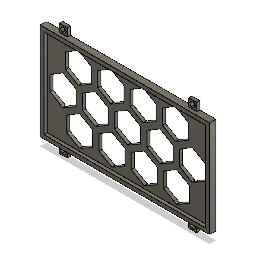
base (Autodesk Fusion 360 design; units mm, degrees)
Autodesk Fusion 360 part; units mm, degrees
sketch "Sketch1" plane through (0, 0, 0) normal (0, 0, 1) x (1, 0, 0)
  line L0 (0, 0) -> (0, 60)
  line L1 (0, 60) -> (10, 60)
  line L2 (10, 60) -> (10, 65)
  line L3 (10, 65) -> (15, 65)
  line L4 (15, 65) -> (15, 60)
  line L5 (15, 60) -> (90, 60)
  line L6 (90, 60) -> (90, 65)
  line L7 (90, 65) -> (95, 65)
  line L8 (95, 65) -> (95, 60)
  line L9 (95, 60) -> (105, 60)
  line L10 (105, 60) -> (105, 0)
  line L11 (105, 0) -> (95, 0)
  line L12 (95, 0) -> (95, -5)
  line L13 (95, -5) -> (90, -5)
  line L14 (90, -5) -> (90, 0)
  line L15 (90, 0) -> (15, 0)
  line L16 (15, 0) -> (15, -5)
  line L17 (15, -5) -> (10, -5)
  line L18 (10, -5) -> (10, 0)
  line L19 (10, 0) -> (0, 0)
  line L20 (10, 60) -> (15, 60) construction
  line L21 (12.5, 60) -> (12.5, 65) construction
  line L22 (90, 60) -> (95, 60) construction
  line L23 (92.5, 60) -> (92.5, 65) construction
  line L24 (90, 0) -> (95, 0) construction
  line L25 (92.5, 0) -> (92.5, -5) construction
  line L26 (10, 0) -> (15, 0) construction
  line L27 (12.5, 0) -> (12.5, -5) construction
  line L28 (13.366, 61) -> (14.2321, 62.5)
  line L29 (14.2321, 62.5) -> (13.366, 64)
  line L30 (13.366, 64) -> (11.634, 64)
  line L31 (11.634, 64) -> (10.7679, 62.5)
  line L32 (10.7679, 62.5) -> (11.634, 61)
  line L33 (11.634, 61) -> (13.366, 61)
  line L34 (94.2321, 62.5) -> (93.366, 64)
  line L35 (93.366, 64) -> (91.634, 64)
  line L36 (91.634, 64) -> (90.7679, 62.5)
  line L37 (90.7679, 62.5) -> (91.634, 61)
  line L38 (91.634, 61) -> (93.366, 61)
  line L39 (93.366, 61) -> (94.2321, 62.5)
  line L40 (94.2321, -2.5) -> (93.366, -1)
  line L41 (93.366, -1) -> (91.634, -1)
  line L42 (91.634, -1) -> (90.7679, -2.5)
  line L43 (90.7679, -2.5) -> (91.634, -4)
  line L44 (91.634, -4) -> (93.366, -4)
  line L45 (93.366, -4) -> (94.2321, -2.5)
  line L46 (13.366, -1) -> (11.634, -1)
  line L47 (11.634, -1) -> (10.7679, -2.5)
  line L48 (10.7679, -2.5) -> (11.634, -4)
  line L49 (11.634, -4) -> (13.366, -4)
  line L50 (13.366, -4) -> (14.2321, -2.5)
  line L51 (14.2321, -2.5) -> (13.366, -1)
  line L52 (2.5, 57.5) -> (102.5, 57.5) construction
  line L53 (102.5, 57.5) -> (102.5, 2.5) construction
  line L54 (102.5, 2.5) -> (2.5, 2.5) construction
  line L55 (2.5, 2.5) -> (2.5, 57.5) construction
  line L56 (2.5, 57.5) -> (0, 57.5) construction
  line L57 (2.5, 57.5) -> (2.5, 60) construction
  line L58 (102.5, 2.5) -> (102.5, 0) construction
  line L59 (102.5, 2.5) -> (105, 2.5) construction
  line L60 (20.2873, 34.6188) -> (12.2873, 39.2376)
  line L61 (12.2873, 39.2376) -> (4.2873, 34.6188)
  line L62 (4.2873, 34.6188) -> (4.2873, 25.3812)
  line L63 (4.2873, 25.3812) -> (12.2873, 20.7624)
  line L64 (12.2873, 20.7624) -> (20.2873, 25.3812)
  line L65 (20.2873, 25.3812) -> (20.2873, 34.6188)
  line L66 (12.2873, 30) -> (12.2873, 57.5) construction
  line L67 (12.2873, 30) -> (12.2873, 2.5) construction
  line L68 (29.8178, 51.3819) -> (21.8178, 56.0007)
  line L69 (21.8178, 56.0007) -> (13.8178, 51.3819)
  line L70 (13.8178, 51.3819) -> (13.8178, 42.1443)
  line L71 (13.8178, 42.1443) -> (21.8178, 37.5255)
  line L72 (21.8178, 37.5255) -> (29.8178, 42.1443)
  line L73 (29.8178, 42.1443) -> (29.8178, 51.3819)
  line L74 (30.5473, 8.7) -> (30.5473, 17.9376)
  line L75 (30.5473, 17.9376) -> (22.5473, 22.5564)
  line L76 (22.5473, 22.5564) -> (14.5473, 17.9376)
  line L77 (14.5473, 17.9376) -> (14.5473, 8.7)
  line L78 (14.5473, 8.7) -> (22.5473, 4.0812)
  line L79 (22.5473, 4.0812) -> (30.5473, 8.7)
  line L80 (21.8178, 34.6188) -> (21.8178, 37.5255) construction
  line L81 (41.8178, 37.5255) -> (49.8178, 42.1443)
  line L82 (49.8178, 42.1443) -> (49.8178, 51.3819)
  line L83 (49.8178, 51.3819) -> (41.8178, 56.0007)
  line L84 (41.8178, 56.0007) -> (33.8178, 51.3819)
  line L85 (33.8178, 51.3819) -> (33.8178, 42.1443)
  line L86 (33.8178, 42.1443) -> (41.8178, 37.5255)
  line L87 (40.2873, 34.6188) -> (32.2873, 39.2376)
  line L88 (32.2873, 39.2376) -> (24.2873, 34.6188)
  line L89 (24.2873, 34.6188) -> (24.2873, 25.3812)
  line L90 (24.2873, 25.3812) -> (32.2873, 20.7624)
  line L91 (32.2873, 20.7624) -> (40.2873, 25.3812)
  line L92 (40.2873, 25.3812) -> (40.2873, 34.6188)
  line L93 (42.5473, 22.5564) -> (34.5473, 17.9376)
  line L94 (50.5473, 17.9376) -> (42.5473, 22.5564)
  line L95 (50.5473, 8.7) -> (50.5473, 17.9376)
  line L96 (42.5473, 4.0812) -> (50.5473, 8.7)
  line L97 (34.5473, 8.7) -> (42.5473, 4.0812)
  line L98 (34.5473, 17.9376) -> (34.5473, 8.7)
  line L99 (61.8178, 37.5255) -> (69.8178, 42.1443)
  line L100 (69.8178, 42.1443) -> (69.8178, 51.3819)
  line L101 (69.8178, 51.3819) -> (61.8178, 56.0007)
  line L102 (61.8178, 56.0007) -> (53.8178, 51.3819)
  line L103 (53.8178, 51.3819) -> (53.8178, 42.1443)
  line L104 (53.8178, 42.1443) -> (61.8178, 37.5255)
  line L105 (60.2873, 34.6188) -> (52.2873, 39.2376)
  line L106 (52.2873, 39.2376) -> (44.2873, 34.6188)
  line L107 (44.2873, 34.6188) -> (44.2873, 25.3812)
  line L108 (44.2873, 25.3812) -> (52.2873, 20.7624)
  line L109 (52.2873, 20.7624) -> (60.2873, 25.3812)
  line L110 (60.2873, 25.3812) -> (60.2873, 34.6188)
  line L111 (62.5473, 22.5564) -> (54.5473, 17.9376)
  line L112 (70.5473, 17.9376) -> (62.5473, 22.5564)
  line L113 (70.5473, 8.7) -> (70.5473, 17.9376)
  line L114 (62.5473, 4.0812) -> (70.5473, 8.7)
  line L115 (54.5473, 8.7) -> (62.5473, 4.0812)
  line L116 (54.5473, 17.9376) -> (54.5473, 8.7)
  line L117 (81.8178, 37.5255) -> (89.8178, 42.1443)
  line L118 (89.8178, 42.1443) -> (89.8178, 51.3819)
  line L119 (89.8178, 51.3819) -> (81.8178, 56.0007)
  line L120 (81.8178, 56.0007) -> (73.8178, 51.3819)
  line L121 (73.8178, 51.3819) -> (73.8178, 42.1443)
  line L122 (73.8178, 42.1443) -> (81.8178, 37.5255)
  line L123 (80.2873, 34.6188) -> (72.2873, 39.2376)
  line L124 (72.2873, 39.2376) -> (64.2873, 34.6188)
  line L125 (64.2873, 34.6188) -> (64.2873, 25.3812)
  line L126 (64.2873, 25.3812) -> (72.2873, 20.7624)
  line L127 (72.2873, 20.7624) -> (80.2873, 25.3812)
  line L128 (80.2873, 25.3812) -> (80.2873, 34.6188)
  line L129 (82.5473, 22.5564) -> (74.5473, 17.9376)
  line L130 (90.5473, 17.9376) -> (82.5473, 22.5564)
  line L131 (90.5473, 8.7) -> (90.5473, 17.9376)
  line L132 (82.5473, 4.0812) -> (90.5473, 8.7)
  line L133 (74.5473, 8.7) -> (82.5473, 4.0812)
  line L134 (74.5473, 17.9376) -> (74.5473, 8.7)
  line L135 (100.2873, 25.3812) -> (100.2873, 34.6188)
  line L136 (100.2873, 34.6188) -> (92.2873, 39.2376)
  line L137 (92.2873, 39.2376) -> (84.2873, 34.6188)
  line L138 (84.2873, 34.6188) -> (84.2873, 25.3812)
  line L139 (84.2873, 25.3812) -> (92.2873, 20.7624)
  line L140 (92.2873, 20.7624) -> (100.2873, 25.3812)
  point P0 (12.5, 62.5)
  point P1 (92.5, 62.5)
  point P2 (92.5, -2.5)
  point P3 (12.5, -2.5)
  point P4 (12.2873, 30)
  point P5 (21.8178, 46.7631)
  point P6 (22.5473, 13.3188)
  dimension "d1" = 60
  dimension "d2" = 5
  dimension "d3" = 5
  dimension "d7" = 105
  dimension "d8" = 10
  dimension "d9" = 1.5
  dimension "d10" = 1.5
  dimension "d11" = 1.5
  dimension "d12" = 1.5
  dimension "d19" = 2.5
  dimension "d21" = 8
  dimension "d29" = -60
  dimension "d30" = 0
  dimension "d33" = 20
  dimension "d34" = 0
  constraint coincident L0.start L19.end
  constraint vertical L0
  constraint perpendicular L0 L1
  constraint perpendicular L1 L2
  constraint perpendicular L2 L3
  constraint perpendicular L3 L4
  constraint perpendicular L4 L5
  constraint perpendicular L5 L6
  constraint perpendicular L4 L7
  constraint perpendicular L7 L8
  constraint perpendicular L8 L9
  constraint perpendicular L7 L10
  constraint perpendicular L10 L11
  constraint perpendicular L11 L12
  constraint perpendicular L12 L13
  constraint perpendicular L13 L14
  constraint perpendicular L14 L15
  constraint perpendicular L15 L16
  constraint perpendicular L16 L17
  constraint perpendicular L15 L18
  constraint perpendicular L0 L19
  constraint equal L3 L7
  constraint equal L7 L13
  constraint equal L13 L17
  constraint equal L1 L19
  constraint equal L11 L19
  constraint equal L9 L11
  constraint equal L2 L6
  constraint equal L6 L14
  constraint equal L14 L16
  constraint equal L4 L8
  constraint equal L2 L4
  constraint equal L2 L18
  constraint equal L12 L18
  constraint midpoint L20 L21.start
  constraint midpoint L3 L21.end
  constraint midpoint L22 L23.start
  constraint midpoint L7 L23.end
  constraint midpoint L24 L25.start
  constraint midpoint L13 L25.end
  constraint midpoint L26 L27.start
  constraint midpoint L17 L27.end
  constraint midpoint L21 P0
  constraint midpoint L23 P1
  constraint midpoint L25 P2
  constraint midpoint L27 P3
  constraint horizontal L46
  constraint horizontal L41
  constraint horizontal L35
  constraint horizontal L30
  constraint horizontal L52
  constraint vertical L53
  constraint horizontal L54
  constraint vertical L55
  constraint coincident L0 L56.end
  constraint perpendicular L0 L56
  constraint coincident L1 L57.end
  constraint perpendicular L1 L57
  constraint coincident L11 L58.end
  constraint perpendicular L11 L58
  constraint coincident L10 L59.end
  constraint perpendicular L10 L59
  constraint equal L56 L57
  constraint equal L56 L59
  constraint equal L58 L59
  constraint coincident P4 L66.start
  constraint coincident L52 L66.end
  constraint perpendicular L52 L66
  constraint coincident L54 L67.end
  constraint perpendicular L54 L67
  constraint equal L66 L67
  constraint vertical L65
  constraint vertical L74
  constraint vertical L73
  constraint equal L60 L71
  constraint equal L71 L76
  constraint vertical L80
  measures "d1" distance of L0.start L0.end
  measures "d2" distance of L2.end L3.end
  measures "d3" distance of L1.end L2.end
  measures "d7" distance of L0.end L9.end
  measures "d8" distance of L0.end L1.end
  measures "d9" distance of P0 L33
  measures "d10" distance of P1 L39
  measures "d11" distance of P2 L45
  measures "d12" distance of P3 L51
  measures "d19" distance of L52.start L56.end
  measures "d21" distance of P4 L65
extrude "Extrude2" add sketch "Sketch1" along normal blind 2
sketch "Sketch2" plane through (0, 0, 0) normal (0, 0, 1) x (1, 0, 0)
  line L0 (0, 0) -> (105, 0)
  line L1 (105, 0) -> (105, 60)
  line L2 (105, 60) -> (0, 60)
  line L3 (0, 60) -> (0, 0)
  line L4 (2.5, 2.5) -> (102.5, 2.5)
  line L5 (102.5, 2.5) -> (102.5, 57.5)
  line L6 (102.5, 57.5) -> (2.5, 57.5)
  line L7 (2.5, 57.5) -> (2.5, 2.5)
  line L8 (2.5, 57.5) -> (0, 57.5) construction
  line L9 (2.5, 57.5) -> (2.5, 60) construction
  line L10 (102.5, 2.5) -> (102.5, 0) construction
  line L11 (102.5, 2.5) -> (105, 2.5) construction
  line L12 (10, 60) -> (0, 60) construction
  line L13 (105, 0) -> (105, 60)
  dimension "d15" = 2.5
  constraint horizontal L0
  constraint vertical L1
  constraint horizontal L2
  constraint vertical L3
  constraint coincident L0.start L3.end
  constraint horizontal L4
  constraint vertical L5
  constraint horizontal L6
  constraint vertical L7
  constraint coincident L3 L8.end
  constraint perpendicular L3 L8
  constraint coincident L2 L9.end
  constraint perpendicular L2 L9
  constraint coincident L0 L10.end
  constraint perpendicular L0 L10
  constraint coincident L1 L11.end
  constraint perpendicular L1 L11
  constraint equal L10 L11
  constraint equal L9 L10
  constraint equal L8 L9
  constraint collinear L2 L12
  constraint collinear L1 L13
  measures "d15" distance of L6.end L8.end
extrude "Extrude3" add sketch "Sketch2" along normal blind 2 from surface at 2
sketch "Sketch3" plane through (0, 0, 0) normal (0, 0, -1) x (-1, 0, 0)
  line L0 (-22.5473, 4.0812) -> (-30.5473, 8.7)
  line L1 (-30.5473, 8.7) -> (-30.5473, 17.9376)
  line L2 (-30.5473, 17.9376) -> (-22.5473, 22.5564)
  line L3 (-22.5473, 22.5564) -> (-14.5473, 17.9376)
  line L4 (-14.5473, 17.9376) -> (-14.5473, 8.7)
  line L5 (-14.5473, 8.7) -> (-22.5473, 4.0812)
  line L6 (-11.634, 61) -> (-13.366, 61)
  line L7 (-13.366, 61) -> (-14.2321, 62.5)
  line L8 (-14.2321, 62.5) -> (-13.366, 64)
  line L9 (-13.366, 64) -> (-11.634, 64)
  line L10 (-11.634, 64) -> (-10.7679, 62.5)
  line L11 (-10.7679, 62.5) -> (-11.634, 61)
  line L12 (-93.366, 61) -> (-94.2321, 62.5)
  line L13 (-94.2321, 62.5) -> (-93.366, 64)
  line L14 (-93.366, 64) -> (-91.634, 64)
  line L15 (-91.634, 64) -> (-90.7679, 62.5)
  line L16 (-90.7679, 62.5) -> (-91.634, 61)
  line L17 (-91.634, 61) -> (-93.366, 61)
  line L18 (-93.366, -4) -> (-94.2321, -2.5)
  line L19 (-94.2321, -2.5) -> (-93.366, -1)
  line L20 (-93.366, -1) -> (-91.634, -1)
  line L21 (-91.634, -1) -> (-90.7679, -2.5)
  line L22 (-90.7679, -2.5) -> (-91.634, -4)
  line L23 (-91.634, -4) -> (-93.366, -4)
  line L24 (-14.2321, -2.5) -> (-13.366, -1)
  line L25 (-13.366, -1) -> (-11.634, -1)
  line L26 (-11.634, -1) -> (-10.7679, -2.5)
  line L27 (-10.7679, -2.5) -> (-11.634, -4)
  line L28 (-11.634, -4) -> (-13.366, -4)
  line L29 (-13.366, -4) -> (-14.2321, -2.5)
  line L30 (-29.8178, 42.1443) -> (-29.8178, 51.3819)
  line L31 (-29.8178, 51.3819) -> (-21.8178, 56.0007)
  line L32 (-21.8178, 56.0007) -> (-13.8178, 51.3819)
  line L33 (-13.8178, 51.3819) -> (-13.8178, 42.1443)
  line L34 (-13.8178, 42.1443) -> (-21.8178, 37.5255)
  line L35 (-21.8178, 37.5255) -> (-29.8178, 42.1443)
  line L36 (-20.2873, 25.3812) -> (-20.2873, 34.6188)
  line L37 (-20.2873, 34.6188) -> (-12.2873, 39.2376)
  line L38 (-12.2873, 39.2376) -> (-4.2873, 34.6188)
  line L39 (-4.2873, 34.6188) -> (-4.2873, 25.3812)
  line L40 (-4.2873, 25.3812) -> (-12.2873, 20.7624)
  line L41 (-12.2873, 20.7624) -> (-20.2873, 25.3812)
  line L42 (-73.8178, 42.1443) -> (-81.8178, 37.5255)
  line L43 (-81.8178, 37.5255) -> (-89.8178, 42.1443)
  line L44 (-89.8178, 42.1443) -> (-89.8178, 51.3819)
  line L45 (-89.8178, 51.3819) -> (-81.8178, 56.0007)
  line L46 (-81.8178, 56.0007) -> (-73.8178, 51.3819)
  line L47 (-73.8178, 51.3819) -> (-73.8178, 42.1443)
  line L48 (-54.5473, 17.9376) -> (-54.5473, 8.7)
  line L49 (-54.5473, 8.7) -> (-62.5473, 4.0812)
  line L50 (-62.5473, 4.0812) -> (-70.5473, 8.7)
  line L51 (-70.5473, 8.7) -> (-70.5473, 17.9376)
  line L52 (-70.5473, 17.9376) -> (-62.5473, 22.5564)
  line L53 (-62.5473, 22.5564) -> (-54.5473, 17.9376)
  line L54 (-60.2873, 25.3812) -> (-60.2873, 34.6188)
  line L55 (-60.2873, 34.6188) -> (-52.2873, 39.2376)
  line L56 (-52.2873, 39.2376) -> (-44.2873, 34.6188)
  line L57 (-44.2873, 34.6188) -> (-44.2873, 25.3812)
  line L58 (-44.2873, 25.3812) -> (-52.2873, 20.7624)
  line L59 (-52.2873, 20.7624) -> (-60.2873, 25.3812)
  line L60 (-53.8178, 42.1443) -> (-61.8178, 37.5255)
  line L61 (-61.8178, 37.5255) -> (-69.8178, 42.1443)
  line L62 (-69.8178, 42.1443) -> (-69.8178, 51.3819)
  line L63 (-69.8178, 51.3819) -> (-61.8178, 56.0007)
  line L64 (-61.8178, 56.0007) -> (-53.8178, 51.3819)
  line L65 (-53.8178, 51.3819) -> (-53.8178, 42.1443)
  line L66 (-34.5473, 17.9376) -> (-34.5473, 8.7)
  line L67 (-34.5473, 8.7) -> (-42.5473, 4.0812)
  line L68 (-42.5473, 4.0812) -> (-50.5473, 8.7)
  line L69 (-50.5473, 8.7) -> (-50.5473, 17.9376)
  line L70 (-50.5473, 17.9376) -> (-42.5473, 22.5564)
  line L71 (-42.5473, 22.5564) -> (-34.5473, 17.9376)
  line L72 (-40.2873, 25.3812) -> (-40.2873, 34.6188)
  line L73 (-40.2873, 34.6188) -> (-32.2873, 39.2376)
  line L74 (-32.2873, 39.2376) -> (-24.2873, 34.6188)
  line L75 (-24.2873, 34.6188) -> (-24.2873, 25.3812)
  line L76 (-24.2873, 25.3812) -> (-32.2873, 20.7624)
  line L77 (-32.2873, 20.7624) -> (-40.2873, 25.3812)
  line L78 (-33.8178, 42.1443) -> (-41.8178, 37.5255)
  line L79 (-41.8178, 37.5255) -> (-49.8178, 42.1443)
  line L80 (-49.8178, 42.1443) -> (-49.8178, 51.3819)
  line L81 (-49.8178, 51.3819) -> (-41.8178, 56.0007)
  line L82 (-41.8178, 56.0007) -> (-33.8178, 51.3819)
  line L83 (-33.8178, 51.3819) -> (-33.8178, 42.1443)
  line L84 (-92.2873, 20.7624) -> (-100.2873, 25.3812)
  line L85 (-100.2873, 25.3812) -> (-100.2873, 34.6188)
  line L86 (-100.2873, 34.6188) -> (-92.2873, 39.2376)
  line L87 (-92.2873, 39.2376) -> (-84.2873, 34.6188)
  line L88 (-84.2873, 34.6188) -> (-84.2873, 25.3812)
  line L89 (-84.2873, 25.3812) -> (-92.2873, 20.7624)
  line L90 (-80.2873, 25.3812) -> (-80.2873, 34.6188)
  line L91 (-80.2873, 34.6188) -> (-72.2873, 39.2376)
  line L92 (-72.2873, 39.2376) -> (-64.2873, 34.6188)
  line L93 (-64.2873, 34.6188) -> (-64.2873, 25.3812)
  line L94 (-64.2873, 25.3812) -> (-72.2873, 20.7624)
  line L95 (-72.2873, 20.7624) -> (-80.2873, 25.3812)
  line L96 (-74.5473, 17.9376) -> (-74.5473, 8.7)
  line L97 (-74.5473, 8.7) -> (-82.5473, 4.0812)
  line L98 (-82.5473, 4.0812) -> (-90.5473, 8.7)
  line L99 (-90.5473, 8.7) -> (-90.5473, 17.9376)
  line L100 (-90.5473, 17.9376) -> (-82.5473, 22.5564)
  line L101 (-82.5473, 22.5564) -> (-74.5473, 17.9376)
  line L102 (-10, -5) -> (-10, 0)
  line L103 (-10, 0) -> (0, 0)
  line L104 (0, 0) -> (0, 60)
  line L105 (0, 60) -> (-10, 60)
  line L106 (-10, 60) -> (-10, 65)
  line L107 (-10, 65) -> (-15, 65)
  line L108 (-15, 65) -> (-15, 60)
  line L109 (-15, 60) -> (-90, 60)
  line L110 (-90, 60) -> (-90, 65)
  line L111 (-90, 65) -> (-95, 65)
  line L112 (-95, 65) -> (-95, 60)
  line L113 (-95, 60) -> (-105, 60)
  line L114 (-105, 60) -> (-105, 0)
  line L115 (-105, 0) -> (-95, 0)
  line L116 (-95, 0) -> (-95, -5)
  line L117 (-95, -5) -> (-90, -5)
  line L118 (-90, -5) -> (-90, 0)
  line L119 (-90, 0) -> (-15, 0)
  line L120 (-15, 0) -> (-15, -5)
  line L121 (-15, -5) -> (-10, -5)
  line L122 (-93.366, 61) -> (-91.634, 61)
  line L123 (-91.634, 61) -> (-91.634, -1)
  line L124 (-91.634, -1) -> (-93.366, -1)
  line L125 (-93.366, -1) -> (-93.366, 61)
  line L126 (-13.366, 61) -> (-11.634, 61)
  line L127 (-11.634, 61) -> (-11.634, -1)
  line L128 (-11.634, -1) -> (-13.366, -1)
  line L129 (-13.366, -1) -> (-13.366, 61)
  constraint coincident L12.start L17.end
  constraint coincident L16.end L17.start
  constraint coincident L20.end L21.start
  constraint coincident L19.end L20.start
  constraint coincident L6.end L7.start
  constraint coincident L6.start L11.end
  constraint coincident L25.end L26.start
  constraint coincident L24.end L25.start
extrude "Extrude4" cut sketch "Sketch3" against normal blind 0.5 contours L6 L37 L38 L126 L127 L129 | L25 L40 L41 L127 L128 L129 | L17 L86 L87 L122 L123 L125 | L20 L84 L89 L123 L124 L125
